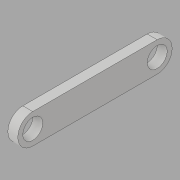
# Autodesk Inventor part: g_connector x4
Saved by Autodesk Inventor 2019 (Build 230136000, 136)
## iProperties
Created: 2021-10-30
Part Number: g_connector x4
Material: Generic
Document SubType Name: Modeling
Designer: Mohamed
Density: 1 g/cm^3
Appearance: Default
Author: Mohamed
Autodesk Inventor part; units mm, degrees
ref_plane "YZ Plane" through (0, 0, 0) normal (1, 0, 0) x (0, 1, 0)
ref_plane "XZ Plane" through (0, 0, 0) normal (0, 1, 0) x (-1, 0, 0)
ref_plane "XY Plane" through (0, 0, 0) normal (0, 0, 1) x (1, 0, 0)
sketch "Sketch1" plane through (0, 0, 0) normal (1, 0, 0) x (0, 1, 0)
  arc A0 (3, 0) -> (-3, 0) centre (0, 0) ccw
  line L0 (3, 0) -> (3, -25)
  arc A1 (-3, -25) -> (3, -25) centre (0, -25) ccw
  line L1 (-3, 0) -> (-3, -25)
  circle A2 centre (0, 0) radius 2
  circle A3 centre (0, -25) radius 2
  dimension "d0" = 6
  dimension "d1" = 25
  dimension "d2" = 6
  dimension "d3" = 4
  dimension "d4" = 4
  constraints: 4 centre point, 4 end point, 4 point on circle, 3 coincident, 1 tangent, 1 vertical
  measures "d0" diameter of A0
  measures "d1" distance of L0.start L0.end
  measures "d2" diameter of A1
  measures "d3" diameter of A2
  measures "d4" diameter of A3
extrude "Extrusion1" add sketch "Sketch1" along normal blind 2
body "Solid1"
